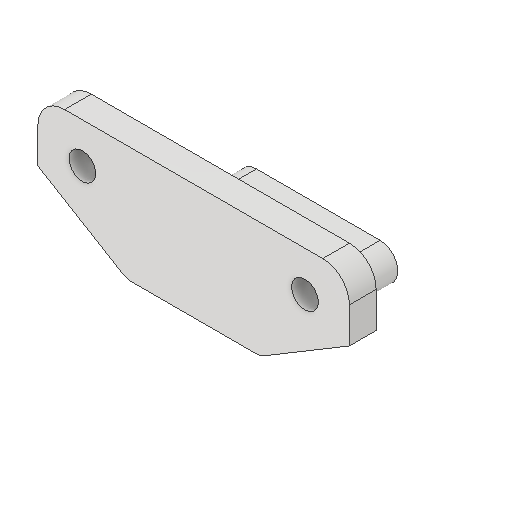
# Autodesk Inventor part: 3DP_PLA_Y_axis_endstop_pushrod
Saved by Autodesk Inventor 2025 (Build 290162010, 162A)
## iProperties
Created: 2018-08-01
Part Number: 3DP_PLA_Y_axis_endstop_pushrod
Material: ABS Plastic
Document SubType Name: Modeling
Designer: Andrzej
Density: 1.06 g/cm^3
Appearance: Smooth - White
Author: Andrzej
Autodesk Inventor part; units mm, degrees
ref_plane "YZ Plane" through (0, 0, 0) normal (1, 0, 0) x (0, 1, 0)
ref_plane "XZ Plane" through (0, 0, 0) normal (0, 1, 0) x (-1, 0, 0)
ref_plane "XY Plane" through (0, 0, 0) normal (0, 0, 1) x (1, 0, 0)
sketch "Sketch1" plane through (0, 0, 0) normal (0, 0, 1) x (1, 0, 0)
  line L0 (-9.4435, 4.8027) -> (25.5565, 4.8027)
  line L1 (25.5565, 4.8027) -> (25.5565, -4.1973)
  line L2 (25.5565, -4.1973) -> (-9.4435, -4.1973)
  line L3 (-9.4435, -4.1973) -> (-9.4435, 4.8027)
  line L4 (-9.4435, -4.1973) -> (-9.4435, -8.1973)
  line L5 (-9.4435, -8.1973) -> (25.5565, -8.1973)
  line L6 (25.5565, -8.1973) -> (25.5565, -4.1973)
  point P0 (0, 0)
  point P1 (-4.4435, 0.3027)
  point P2 (20.5565, 0.3027)
  dimension "d0" = 35
  dimension "d1" = 9
  dimension "d2" = 25
  dimension "d3" = 5
  dimension "d4" = 4.5
  dimension "d5" = 4
  constraints: 14 end point, 3 perpendicular, 2 parallel, 1 horizontal, 1 horizontal alignment, 1 vertical
  measures "d0" distance of L1.end L2.end
  measures "d1" distance of L0.end L1.end
  measures "d2" distance of point (20.557, 0.303) point (-4.443, 0.303)
  measures "d3" distance from line of L1 point (20.557, 0.303)
  measures "d4" distance from line of L2 point (20.557, 0.303)
  measures "d5" distance between parallel lines of L2 L5
extrude "Extrusion1" add sketch "Sketch1" along normal blind 3
extrude "Extrusion2" add sketch "Sketch1" against normal blind 11 contours L2 L6 L5 L4
hole "Hole1" at (-4.4435, 0.3027, 0) at (20.5565, 0.3027, 0) direction (0, 0, 1) diameter 3 end through all
fillet "Fillet1" radius 3 2 edges at (-9.4435, 4.8027, 1.5) (25.5565, 4.8027, 1.5)
chamfer "Chamfer1" distance 6 distance2 10 1 edges at (-9.4435, -8.1973, -4) measured on face at (-9.4435, -7.6973, -4)
chamfer "Chamfer2" distance 6 distance2 10 1 edges at (25.5565, -8.1973, -4) measured on face at (25.5565, -7.6973, -4)
fillet "Fillet2" radius 2 4 edges at (22.2232, -4.1973, -5.5) (-6.1102, -4.1973, -5.5) (0.5565, -8.1973, -4) (15.5565, -8.1973, -4)
sketch "Sketch2" plane through (0, 0, -11) normal (0, 0, -1) x (-1, 0, 0)
  arc A0 (-15.0025, -4.1973) -> (-15.0025, -8.1973) centre (-15.0025, -6.1973) ccw projected
  line L0 (-15.0025, -8.1973) -> (-1.1105, -8.1973) projected
  arc A1 (-1.1105, -8.1973) -> (-1.1105, -4.1973) centre (-1.1105, -6.1973) ccw projected
  line L1 (-1.1105, -4.1973) -> (-15.0025, -4.1973) projected
  line L2 (-15.0025, -8.1973) -> (-1.1105, -8.1973) projected
  line L3 (-3.0565, -8.1973) -> (-3.0565, -16.1973)
  line L4 (-3.0565, -16.1973) -> (-13.0565, -16.1973)
  line L5 (-13.0565, -16.1973) -> (-13.0565, -8.1973)
  point P0 (0, 0)
  dimension "d25" = 8
  dimension "d26" = 10
  dimension "d27" = 13.8921
  dimension "d28" = 1.946
  constraints: 6 end point, 3 perpendicular, 2 point on line
  measures "d25" distance between parallel lines of L0 L4
  measures "d26" distance between parallel lines of L5 L3
  measures "d27" distance of A0.centre A1.centre
  measures "d28" distance from line of A1.centre L3
extrude "Extrusion3" add sketch "Sketch2" against normal blind 3 contours L0 L3 L4 L5
chamfer "Chamfer3" distance 8 distance2 3 1 edges at (3.0565, -16.1973, -9.5) measured on face at (3.0565, -15.6973, -9.5)
chamfer "Chamfer4" distance 8 distance2 3 1 edges at (13.0565, -16.1973, -9.5) measured on face at (13.0565, -15.6973, -9.5)
fillet "Fillet3" radius 2 2 edges at (10.0566, -16.1973, -9.5) (6.0564, -16.1973, -9.5)
equation "\"d1\" = 2 * d4"
equation "\"d28\" = -0.5 * d26 + 0.5 * d27"
body "Solid1"
